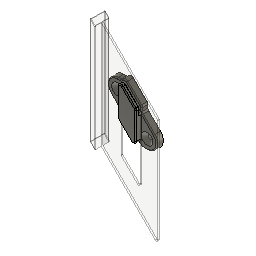
model (Autodesk Fusion 360 design; units mm, degrees)
Autodesk Fusion 360 part; units mm, degrees
sketch "Sketch1" plane through (0, 0, 0) normal (0, 1, 0) x (1, 0, 0)
  line L0 (62.4, 0) -> (0, -62.4)
  line L1 (0, -62.4) -> (0, -171.4)
  line L2 (0, -171.4) -> (62.4, -109)
  line L3 (62.4, -109) -> (62.4, 0)
  line L4 (4.9, -166.5) -> (4.9, -57.5)
  line L5 (25, -124.4797) -> (44.3, -105.1797)
  line L6 (44.3, -105.1797) -> (44.3, -40.3032)
  line L7 (44.3, -40.3032) -> (25, -59.6032)
  line L8 (25, -59.6032) -> (25, -124.4797)
  line L9 (0, 0) -> (62.4, 0) construction
  line L10 (0, -62.4) -> (0, 0) construction
  dimension "d1" = 62.4
  dimension "d2" = 45
  dimension "d3" = 109
  dimension "d4" = 4.9
  dimension "d5" = 18.1
  dimension "d6" = 15.5
  dimension "d7" = 15.7
  dimension "d8" = 25
  constraint vertical L1
  constraint vertical L3
  constraint parallel L0 L2
  constraint coincident L2 L4.start
  constraint coincident L0 L4.end
  constraint vertical L4
  constraint vertical L6
  constraint vertical L8
  constraint parallel L5 L7
  constraint parallel L2 L5
  constraint coincident L9.start L10.end
  constraint horizontal L9
  constraint vertical L10
  measures "d1" horizontal distance of L0.start L0.end
  measures "d2" angle of L0 L3
  measures "d3" distance of L0.start L2.end
  measures "d4" horizontal distance of L0.end L4.end
  measures "d5" distance of L3 L6
  measures "d6" distance of L2 L5
  measures "d7" distance of L0 L7
  measures "d8" distance of L1 L8
extrude "Extrude1" add sketch "Sketch1" along normal mid plane 1.75 contours L0 L2 L3 L4 makes body 1
extrude "Extrude2" add sketch "Sketch1" along normal mid plane 14.8 contours L0 L1 L2 L4 bodies 1
fillet "Fillet1" radius 0.5 7 edges at (0, 0, 171.4) (0, 0, 62.4) (62.4, 0, 109) (44.3, 0, 105.1797) (25, 0, 59.6032) (4.9, 4.1375, 166.5) (4.9, -4.1375, 166.5) 2 faces at (3.2667, -7.4, 95.4667) (3.2667, 7.4, 95.4667) on bodies 1
fillet "Fillet2" radius 1.5 3 edges at (25, 0, 124.4797) (44.3, 0, 40.3032) (62.4, 0, 0) on bodies 1
sketch "Sketch2" plane through (0, -0.875, 0) normal (0, -1, 0) x (1, 0, 0)
  line L0 (25, 59.8103) -> (25, 120.8584)
  arc A0 (27.5607, 121.919) -> (25, 120.8584) centre (26.5, 120.8584) ccw
  line L1 (27.5607, 121.919) -> (44.1536, 105.3261)
  arc A1 (44.3, 104.9726) -> (44.1536, 105.3261) centre (43.8, 104.9726) ccw
  line L2 (44.3, 104.9726) -> (44.3, 43.9245)
  arc A2 (41.7393, 42.8638) -> (44.3, 43.9245) centre (42.8, 43.9245) ccw
  line L3 (41.7393, 42.8638) -> (25.1464, 59.4567)
  arc A3 (25, 59.8103) -> (25.1464, 59.4567) centre (25.5, 59.8103) ccw
  arc A4 (59.8393, 2.5607) -> (62.4, 3.6213) centre (60.9, 3.6213) ccw
  line L4 (62.4, 3.6213) -> (62.4, 108.7929)
  arc A5 (62.4, 108.7929) -> (62.2536, 109.1464) centre (61.9, 108.7929) ccw
  line L5 (62.2536, 109.1464) -> (4.7536, 166.6464)
  arc A6 (4.9, 166.2929) -> (4.7536, 166.6464) centre (4.4, 166.2929) ccw
  line L6 (4.9, 166.2929) -> (4.9, 57.5)
  line L7 (4.9, 57.5) -> (59.8393, 2.5607)
  line L8 (25.25, 94.6198) -> (25.25, 129.8865)
  line L9 (25.25, 129.8865) -> (44.05, 111.0865)
  line L10 (44.05, 111.0865) -> (44.05, 75.8198)
  line L11 (25.25, 94.6198) -> (44.05, 75.8198)
  line L12 (34.65, 120.4865) -> (34.65, 85.2198) construction
  line L13 (34.65, 85.2198) -> (34.65, 49.9532) construction
  circle A7 centre (19.5, 114.3466) radius 2.25
  circle A8 centre (19.5, 114.3466) radius 5.75 construction
  line L14 (25.25, 94.6198) -> (12.5116, 107.3582)
  arc A9 (19.5, 124.2297) -> (12.5116, 107.3582) centre (19.5, 114.3466) ccw
  line L15 (19.5, 124.2297) -> (25.25, 124.2297)
  line L16 (49.8, 75.8198) -> (44.05, 75.8198)
  line L17 (44.05, 105.4297) -> (56.7884, 92.6913)
  arc A10 (49.8, 75.8198) -> (56.7884, 92.6913) centre (49.8, 85.7029) ccw
  circle A11 centre (49.8, 85.7029) radius 2.25
  point P0 (34.65, 100.0248)
  dimension "d17" = 0.25
  dimension "d18" = 0.25
  dimension "d19" = 4
  dimension "d20" = 4.5
  dimension "d21" = 11.5
  dimension "d23" = 360
  constraint vertical L8
  constraint vertical L10
  constraint parallel L1 L9
  constraint equal L8 L10
  constraint midpoint L9 L12.start
  constraint midpoint L11 L12.end
  constraint coincident L3 L13.end
  constraint vertical L13
  constraint equal L12 L13
  constraint concentric A7 A8
  constraint tangent L14 A9
  constraint coincident L8 L15.end
  constraint tangent A9 L15
  constraint coincident A7.centre A8.centre
  constraint collinear L11 L14
  constraint tangent L8 A8
  constraint horizontal L15
  constraint coincident L12 P0
  constraint coincident L10.end L11.end
  constraint coincident L1 L17.start
  measures "d17" distance of L0 L8
  measures "d18" distance of L2 L10
  measures "d19" distance of L1 L9
  measures "d20" diameter of A7
  measures "d21" diameter of A8
extrude "Extrude3" add sketch "Sketch2" against normal up to surface (1.75 mm away) separate body contours A0 L1 L8 L10 L11 makes body 2
extrude "Extrude4" add sketch "Sketch2" against normal up to surface (6.525 mm away) from surface at -1.75 contours L0 A0 L8 L14 A9 L15 | L0 A0 L8 L14 | A0 L1 L8 L10 L11 | A0 L1 L8 L9 L10 | L1 A1 L2 L10 L16 L17 | A1 L2 L16 L17 A10 bodies 2
extrude "Extrude5" add sketch "Sketch2" along normal blind 4 contours A0 L1 L8 L10 L11 | A0 L1 L8 L9 L10 bodies 2
chamfer "Chamfer1" distance 3.5 angle 45 2 edges at (17.4023, 0.875, 115.1603) (47.7023, 0.875, 86.5166) on bodies 2
fillet "Fillet3" radius 3 11 edges at (25.25, -2, 94.6198) (44.05, -2, 75.8198) (44.05, 4.1375, 75.8198) (44.05, -2.875, 111.0865) (44.05, 4.1375, 111.0865) (25.25, -2.875, 129.8865) (25.25, 4.1375, 129.8865) (25.25, 0, 121.6875) (44.05, 0, 105.4297) (44.05, 4.1375, 105.4297) (25.25, 4.1375, 124.2297) on bodies 2
chamfer "Chamfer2" distance 1 angle 45 25 edges at (10.3692, 0.875, 118.1287) (19.3201, 0.875, 100.5497) (20.875, 0.875, 124.2297) (36.2165, 0.875, 118.92) (26.8895, 0.875, 126.743) (44.05, 0.875, 108.2581) (43.8216, 0.875, 110.992) (36.7713, -0.875, 118.3652) (43.8216, -0.875, 110.992) (44.05, -0.875, 107.0155) (25.25, -0.875, 119.8155) (27.1019, -0.875, 125.4155) (50.4192, 0.875, 99.0605) (41.05, 0.875, 78.8198) (44.1446, 0.875, 76.0482) (47.5463, 0.875, 75.8198) (58.9308, 0.875, 81.9208) (44.05, -4.875, 96.4532) (43.8216, -4.875, 110.992) (36.7713, -4.875, 118.3652) (27.1019, -4.875, 125.4155) (25.25, -4.875, 109.2532) (25.4784, -4.875, 94.7144) (32.5287, -4.875, 87.3412) (42.1981, -4.875, 80.2909) on bodies 2
equation "d18 = d17"
